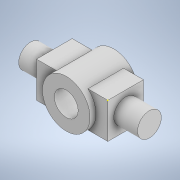
# Autodesk Inventor part: 12
Saved by Autodesk Inventor 2022 (Build 260153000, 153)
## iProperties
Created: 2022-03-14
Part Number: 12
Material: Všeobecné
Document SubType Name: Modeling
Designer: Šimon
Density: 1 g/cm^3
Appearance: Výchozí
Author: Šimon
Autodesk Inventor part; units mm, degrees
ref_plane "YZ Plane" through (0, 0, 0) normal (1, 0, 0) x (0, 1, 0)
ref_plane "XZ Plane" through (0, 0, 0) normal (0, 1, 0) x (-1, 0, 0)
ref_plane "XY Plane" through (0, 0, 0) normal (0, 0, 1) x (1, 0, 0)
sketch "Náčrt1" plane through (0, 0, 0) normal (0, 0, 1) x (1, 0, 0)
  point P0 (0, 0)
sketch "Náčrt2" plane through (0, 0, 0) normal (0, 0, 1) x (1, 0, 0)
  point P0 (0, 0)
sketch "Náčrt3" plane through (0, 0, 0) normal (1, 0, 0) x (0, 1, 0)
  line L0 (0, 0) -> (-30, 0)
  line L1 (-30, 0) -> (-30, -30)
  line L2 (-30, -30) -> (0, -30)
  line L3 (0, -30) -> (0, 0)
  dimension "d0" = 30
  dimension "d1" = 30
  constraints: 8 end point, 2 parallel, 1 horizontal, 1 perpendicular
  measures "d0" distance of L2.end L1.end
  measures "d1" distance of L1.end L0.end
extrude "Vysunutí1" add sketch "Náčrt3" against normal blind 60
sketch "Náčrt4" plane through (0, -30, 0) normal (0, 0, 1) x (1, 0, 0)
  circle A0 centre (-30, 15) radius 20
  point P0 (0, 30)
  dimension "d4" = 40
  constraints: 1 centre point
  measures "d4" diameter of A0
extrude "Vysunutí2" add sketch "Náčrt4" along normal blind 5 and the other way blind 35
sketch "Náčrt5" plane through (-30, -15, 5) normal (0, 0, 1) x (1, 0, 0)
  circle A0 centre (0, 0) radius 10
  point P0 (30, 15)
  dimension "d9" = 20
  constraints: 1 centre point
  measures "d9" diameter of A0
extrude "Vysunutí3" cut sketch "Náčrt5" against normal through all
sketch "Náčrt6" plane through (0, 0, 0) normal (1, 0, 0) x (0, 0, -1)
  circle A0 centre (15, -15) radius 10
  point P0 (0, 0)
  dimension "d12" = 20
  constraints: 1 centre point
  measures "d12" diameter of A0
extrude "Vysunutí4" add sketch "Náčrt6" along normal blind 20
sketch "Náčrt7" plane through (-60, 0, 0) normal (-1, 0, 0) x (0, 0, 1)
  circle A0 centre (-15, -15) radius 10
  point P0 (0, 0)
  dimension "d15" = 20
  constraints: 1 centre point
  measures "d15" diameter of A0
extrude "Vysunutí5" add sketch "Náčrt7" along normal blind 20
